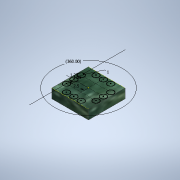
# Autodesk Inventor part: sensor_unit
Saved by Autodesk Inventor 2022.3 (Build 263350000, 350)
## iProperties
Created: 2022-07-18
Part Number: sensor_unit
Material: Generic
Document SubType Name: Modeling
Designer: swang
Density: 1 g/cm^3
Appearance: Default
Author: swang
Autodesk Inventor part; units mm, degrees
ref_plane "YZ Plane" through (0, 0, 0) normal (1, 0, 0) x (0, 1, 0)
ref_plane "XZ Plane" through (0, 0, 0) normal (0, 1, 0) x (-1, 0, 0)
ref_plane "XY Plane" through (0, 0, 0) normal (0, 0, 1) x (1, 0, 0)
sketch "Sketch1" plane through (0, 0, 0) normal (0, 1, 0) x (-1, 0, 0)
  line L0 (-3.1, -3.1) -> (3.1, -3.1)
  line L1 (3.1, -3.1) -> (3.1, 3.1)
  line L2 (3.1, 3.1) -> (-3.1, 3.1)
  line L3 (-3.1, 3.1) -> (-3.1, -3.1)
  line L4 (-3.1, -3.1) -> (3.1, 3.1) construction
  line L5 (3.1, -3.1) -> (-3.1, 3.1) construction
  point P0 (0, 0)
  dimension "d0" = 6
  dimension "d1" = 6
  constraints: 12 end point, 2 midpoint, 2 parallel, 1 horizontal, 1 perpendicular
extrude "Extrusion1" add sketch "Sketch1" along normal blind 1.6
sketch "Sensing Face" plane through (0, 1.6, 0) normal (0, 1, 0) x (1, 0, 0)
  circle A0 centre (-2.5, 1.25) radius 0.5
  line L0 (3.1, 3.1) -> (-3.1, 3.1) construction
  line L1 (0, 3.1) -> (0, -3.1) construction
  line L2 (-3.1, -3.1) -> (3.1, -3.1) construction
  circle A1 centre (-2.5, 0) radius 0.5
  circle A2 centre (-2.5, -1.25) radius 0.5
  circle A3 centre (-1.25, -2.5) radius 0.5
  circle A4 centre (0, -2.5) radius 0.5
  circle A5 centre (1.25, -2.5) radius 0.5
  circle A6 centre (2.5, -1.25) radius 0.5
  circle A7 centre (2.5, 0) radius 0.5
  circle A8 centre (2.5, 1.25) radius 0.5
  circle A9 centre (1.25, 2.5) radius 0.5
  circle A10 centre (0, 2.5) radius 0.5
  circle A11 centre (-1.25, 2.5) radius 0.5
  line L3 (-2.5, 1.25) -> (2.5, 1.25) construction
  line L4 (-2.5, 0) -> (2.5, 0) construction
  line L5 (-2.5, -1.25) -> (2.5, -1.25) construction
  point P0 (0, 0)
  dimension "d4" = 1
  dimension "d5" = 1.25
  dimension "d6" = 2.5
  dimension "d9" = 1.25
  dimension "d16" = 360
  dimension "d20" = 1.25
  constraints: 12 centre point, 8 end point, 2 midpoint, 2 vertical, 35 other
  measures "d4" diameter of A0
  measures "d5" vertical distance of point (0, 0) L3.start
  measures "d6" horizontal distance of point (0, 0) L3.start
  measures "d9" distance of L3.start A1.centre
  measures "d20" distance of L3.start L4.start
equation "\"d1\" = d0"
body "Solid1"
